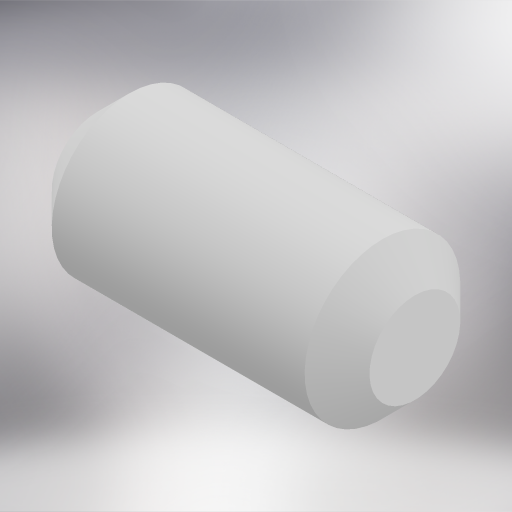
# Autodesk Inventor part: joint_white_part_1
Saved by Autodesk Inventor 2024 (Build 280153000, 153)
## iProperties
Created: 2023-10-25
Part Number: joint_white_part_1
Material: Generic
Document SubType Name: Modeling
Designer: SSAFY
Density: 1 g/cm^3
Appearance: Default
Author: SSAFY
Autodesk Inventor part; units mm, degrees
ref_plane "YZ Plane" through (0, 0, 0) normal (1, 0, 0) x (0, 1, 0)
ref_plane "XZ Plane" through (0, 0, 0) normal (0, 1, 0) x (-1, 0, 0)
ref_plane "XY Plane" through (0, 0, 0) normal (0, 0, 1) x (1, 0, 0)
sketch "Sketch1" plane through (0, 0, 0) normal (0, 0, 1) x (1, 0, 0)
  line L0 (0, 0) -> (-9.8, 0)
  line L1 (-9.8, 0) -> (-9.8, 2.4)
  line L2 (-9.8, 2.4) -> (0, 2.4)
  line L3 (0, 2.4) -> (0, 0)
  point P0 (-4.9, 0)
  dimension "d0" = 9.8
  dimension "d1" = 4.8
  constraints: 8 end point, 2 parallel, 1 horizontal, 1 midpoint, 1 perpendicular
  measures "d0" distance of L1.end L2.end
  measures "d1" diameter of L2 point (-4.9, 0)
revolve "Revolution1" add sketch "Sketch1" angle 360 about axis through (0, 0, 0) along (-1, 0, 0)
chamfer "Chamfer1" distance 1 angle 45 2 edges at (-9.8, -2.4, 0) (0, -2.4, 0)
body "Solid1"
